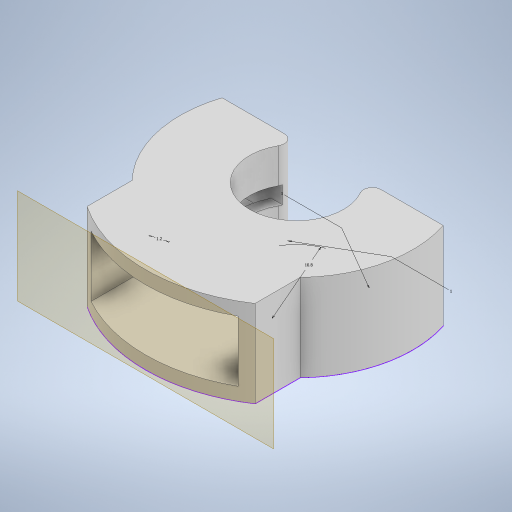
# Autodesk Inventor part: ir다이오드(최종으로가는과정)
Saved by Autodesk Inventor 2023 (Build 270158000, 158)
## iProperties
Created: 2023-04-25
Part Number: ir다이오드(최종으로가는과정)
Material: 일반
Document SubType Name: Modeling
Designer: rlatk
Density: 1 g/cm^3
Appearance: 기본값
Author: rlatk
Autodesk Inventor part; units mm, degrees
ref_plane "YZ Plane" through (0, 0, 0) normal (1, 0, 0) x (0, 1, 0)
ref_plane "XZ Plane" through (0, 0, 0) normal (0, 1, 0) x (-1, 0, 0)
ref_plane "XY Plane" through (0, 0, 0) normal (0, 0, 1) x (1, 0, 0)
sketch "스케치1" plane through (0, 0, 0) normal (0, 1, 0) x (-1, 0, 0)
  arc A0 (4.6935, -2.6705) -> (-4.6935, -2.6705) centre (0, 0) ccw
  arc A1 (12.7363, -4.165) -> (9.6775, 9.2685) centre (0, 0) ccw
  arc A2 (-9.6775, 9.2685) -> (-12.7363, -4.165) centre (0, 0) ccw
  line L0 (12.7363, -4.165) -> (5.5626, -4.165)
  line L1 (-5.5626, -4.165) -> (-12.7363, -4.165)
  arc A3 (4.6935, -2.6705) -> (5.5626, -4.165) centre (5.5626, -3.165) ccw
  arc A4 (-5.5626, -4.165) -> (-4.6935, -2.6705) centre (-5.5626, -3.165) ccw
  arc A5 (9.6775, 14.4605) -> (-9.6775, 14.4605) centre (0, 0) ccw
  line L2 (9.6775, 9.2685) -> (9.6775, 14.4605)
  line L3 (-9.6775, 9.2685) -> (-9.6775, 14.4605)
  arc A6 (11.8342, -2.965) -> (8.4775, 8.7734) centre (0, 0) ccw
  line L4 (11.8342, -2.965) -> (5.8965, -2.965)
  arc A7 (5.8965, -2.965) -> (-5.8965, -2.965) centre (0, 0) ccw
  line L5 (-5.8965, -2.965) -> (-11.8342, -2.965)
  arc A8 (-8.4775, 8.7734) -> (-11.8342, -2.965) centre (0, 0) ccw
  line L6 (-8.4775, 8.7734) -> (-8.4775, 13.8048)
  line L7 (8.4775, 13.8048) -> (8.4775, 8.7734)
  line L8 (-8.4775, 13.8048) -> (-8.4775, 15.1951)
  line L9 (8.4775, 13.8048) -> (8.4775, 15.1951)
  line L10 (5.8965, -2.965) -> (4.5828, -2.965)
  line L11 (-5.8965, -2.965) -> (-4.5828, -2.965)
  point P0 (0, 11.4)
  point P1 (-3.4369, -4.165)
  point P2 (3.4369, -4.165)
  dimension "d42" = 10.8
  dimension "d46" = 1
  dimension "d47" = 1
  dimension "d48" = 1.2
  constraints: 24 end point, 24 point on circle, 9 centre point, 4 tangent, 3 coincident, 3 horizontal, 3 parallel, 3 point on line, 1 vertical, 5 other
  measures "d42" diameter of A0
  measures "d46" radius of A3
  measures "d47" radius of A4
  measures "d48" radial gap between concentric circles of A1 A6
extrude "돌출15" add sketch "스케치1" along normal blind 10
extrude "돌출16" cut sketch "스케치1" along normal blind 7.5 contours A7 L5 A8 L6 L8 A5 L9 L7 A6 L4
extrude "돌출17" add sketch "스케치1" along normal blind 2.5 contours A7 L5 A8 L6 L8 A5 L9 L7 A6 L4
ref_plane "작업 평면3" through (0, 0, 17.4) normal (0, 0, 1) x (1, 0, 0)
sketch "스케치6" plane through (0, 0, 17.4) normal (0, 0, 1) x (1, 0, 0)
  line L0 (8.4775, 8.5) -> (-8.4775, 8.5)
  line L1 (-8.4775, 8.5) -> (-8.4775, 1.5)
  line L2 (-8.4775, 1.5) -> (8.4775, 1.5)
  line L3 (8.4775, 1.5) -> (8.4775, 8.5)
  line L4 (8.4775, 7.5) -> (-8.4775, 7.5) projected
  line L5 (8.4775, 2.5) -> (-8.4775, 2.5) projected
  point P0 (0, 0)
  dimension "d55" = 1
  dimension "d56" = 1
  constraints: 8 end point, 2 parallel, 1 horizontal, 1 perpendicular
  measures "d55" distance between parallel lines of L0 L4
  measures "d56" distance between parallel lines of L2 L5
extrude "돌출18" cut sketch "스케치6" against normal blind 11
extrude "돌출19" cut sketch "스케치1" along normal blind 6 contours A0 A4 L11 A7 L10 A3
extrude "돌출20" add sketch "스케치1" along normal blind 4 contours A0 A4 L11 A7 L10 A3
